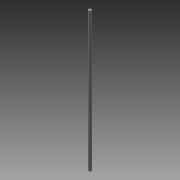
# Autodesk Inventor part: SuperHexagon
Saved by Autodesk Inventor 2013 (Build 170138000, 138)
## iProperties
Created: 2014-01-21
Part Number: SuperHexagon
Material: Generic
Document SubType Name: Modeling
Designer: RobertB
Density: 1 g/cm^3
Author: RobertB
Autodesk Inventor part; units mm, degrees
ref_plane "YZ Plane" through (0, 0, 0) normal (1, 0, 0) x (0, 1, 0)
ref_plane "XZ Plane" through (0, 0, 0) normal (0, 1, 0) x (-1, 0, 0)
ref_plane "XY Plane" through (0, 0, 0) normal (0, 0, 1) x (1, 0, 0)
sketch "Sketch1" plane through (0, 0, 0) normal (0, 1, 0) x (-1, 0, 0)
  circle A0 centre (0, 0) radius 6.35
  line L0 (3.1132, 5.5345) -> (6.3496, 0.0712)
  line L1 (6.3496, 0.0712) -> (3.2364, -5.4633)
  line L2 (3.2364, -5.4633) -> (-3.1132, -5.5345)
  line L3 (-3.1132, -5.5345) -> (-6.3496, -0.0712)
  line L4 (-6.3496, -0.0712) -> (-3.2364, 5.4633)
  line L5 (-3.2364, 5.4633) -> (3.1132, 5.5345)
  dimension "d0" = 12.7
  constraints: 12 end point, 2 coincident, 16 other
extrude "Extrusion1" add sketch "Sketch1" along normal blind 577.85 contours L1 L2 L3 L4 L5 L0
body "Solid1"
